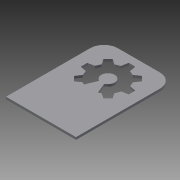
# Autodesk Inventor part: VerticalPiece
Saved by Autodesk Inventor 2014 SP1 (Build 180222100, 222)
## iProperties
Created: 2015-01-04
Part Number: VerticalPiece
Material: Generic
Document SubType Name: Modeling
Designer: Erin
Density: 1 g/cm^3
Appearance: Default
Author: Erin
Autodesk Inventor part; units mm, degrees
ref_plane "YZ Plane" through (0, 0, 0) normal (1, 0, 0) x (0, 1, 0)
ref_plane "XZ Plane" through (0, 0, 0) normal (0, 1, 0) x (-1, 0, 0)
ref_plane "XY Plane" through (0, 0, 0) normal (0, 0, 1) x (1, 0, 0)
sketch "Sketch1" plane through (0, 0, 0) normal (0, 0, 1) x (1, 0, 0)
  line L0 (-15, -18) -> (15, -18)
  line L1 (15, -18) -> (15, 18)
  line L2 (9, 24) -> (-9, 24)
  line L3 (-15, 18) -> (-15, -18)
  arc A0 (-9, 24) -> (-15, 18) centre (-9, 18) ccw
  arc A1 (15, 18) -> (9, 24) centre (9, 18) ccw
  point P0 (0, 0)
  point P1 (15, 24)
  point P2 (-15, 24)
  point P3 (15, 0)
  point P4 (0, 24)
  dimension "d0" = 30
  dimension "d1" = 42
  dimension "d2" = 6
  constraints: 8 end point, 4 point on circle, 4 point on line, 4 tangent, 2 centre point, 2 midpoint, 2 parallel, 1 equal radius, 1 horizontal, 1 horizontal alignment, 1 perpendicular, 1 vertical alignment
  measures "d0" distance of point (-15, 24) point (15, 24)
  measures "d1" distance of point (15, 24) L0.end
  measures "d2" radius of A0
extrude "Extrusion1" add sketch "Sketch1" along normal blind 1
sketch "Sketch2" plane through (0, 0, 0) normal (0, 0, 1) x (1, 0, 0)
  arc A0 (-3.8619, 17.3067) -> (-3.6654, 17.2925) centre (-3.7499, 17.4911) ccw
  line L0 (-3.6654, 17.2925) -> (-1.9114, 18.0105)
  arc A1 (-1.9114, 18.0105) -> (-1.782, 18.1586) centre (-1.9892, 18.209) ccw
  line L1 (-1.782, 18.1586) -> (-1.2951, 20.7754)
  arc A2 (-1.1603, 20.8876) -> (-1.2951, 20.7754) centre (-1.1555, 20.7447) ccw
  line L2 (-1.1603, 20.8876) -> (0.1418, 20.8876)
  arc A3 (3.0232, 10.5703) -> (-2.7384, 10.57) centre (0.1424, 10.5701) ccw
  arc A4 (-2.7384, 10.57) -> (-1.4094, 8.1444) centre (0.1397, 10.5701) ccw
  arc A5 (-1.4094, 8.1444) -> (-1.2693, 8.0371) centre (-0.717, 8.9031) ccw
  line L3 (-1.2693, 8.0371) -> (-1.0511, 7.9035)
  line L4 (-0.9944, 7.7366) -> (-2.8191, 3.3275)
  arc A6 (-2.9648, 3.2741) -> (-2.8191, 3.3275) centre (-2.9158, 3.3658) ccw
  line L5 (-2.9648, 3.2741) -> (-3.8472, 3.7453)
  arc A7 (-3.8472, 3.7453) -> (-4.0418, 3.7399) centre (-3.9398, 3.572) ccw
  line L6 (-4.0418, 3.7399) -> (-6.0484, 2.3626)
  arc A8 (-6.2232, 2.3788) -> (-6.0484, 2.3626) centre (-6.1253, 2.4841) ccw
  line L7 (-6.2232, 2.3788) -> (-8.061, 4.2166)
  arc A9 (-8.0807, 4.3951) -> (-8.061, 4.2166) centre (-7.9596, 4.3181) ccw
  line L8 (-8.0807, 4.3951) -> (-6.6787, 6.4378)
  arc A10 (-6.6787, 6.4378) -> (-6.6624, 6.6306) centre (-6.8628, 6.5504) ccw
  line L9 (-6.6624, 6.6306) -> (-7.436, 8.5631)
  arc A11 (-7.436, 8.5631) -> (-7.581, 8.6886) centre (-7.6302, 8.4854) ccw
  line L10 (-7.581, 8.6886) -> (-10.0488, 9.1479)
  arc A12 (-10.161, 9.2831) -> (-10.0488, 9.1479) centre (-10.0181, 9.2876) ccw
  line L11 (-10.161, 9.2831) -> (-10.1612, 11.8869)
  arc A13 (-10.049, 12.0221) -> (-10.1612, 11.8869) centre (-10.018, 11.8822) ccw
  line L12 (-10.049, 12.0221) -> (-7.5191, 12.4926)
  arc A14 (-7.5191, 12.4926) -> (-7.3693, 12.6214) centre (-7.5703, 12.7036) ccw
  line L13 (-7.3693, 12.6214) -> (-6.5937, 14.4306)
  arc A15 (-6.5937, 14.4306) -> (-6.6058, 14.6262) centre (-6.7865, 14.5168) ccw
  line L14 (-6.6058, 14.6262) -> (-8.0801, 16.7747)
  arc A16 (-8.0639, 16.9496) -> (-8.0801, 16.7747) centre (-7.9592, 16.8517) ccw
  line L15 (-8.0639, 16.9496) -> (-6.2228, 18.7908)
  arc A17 (-6.048, 18.8069) -> (-6.2228, 18.7908) centre (-6.125, 18.6867) ccw
  line L16 (-6.048, 18.8069) -> (-3.8619, 17.3067)
  arc A18 (-0.9944, 7.7366) -> (-1.0511, 7.9035) centre (-1.1231, 7.786) ccw
  line L17 (0.1418, 20.8876) -> (0.1429, 2.0479) construction
  arc A19 (2.0659, 18.1588) -> (2.1953, 18.0107) centre (2.2731, 18.2093) ccw
  line L18 (2.0659, 18.1588) -> (1.5788, 20.7755)
  arc A20 (1.6945, 8.1446) -> (3.0232, 10.5703) centre (0.145, 10.5701) ccw
  arc A21 (1.5544, 8.0373) -> (1.6945, 8.1446) centre (1.002, 8.9032) ccw
  line L19 (1.5544, 8.0373) -> (1.3362, 7.9037)
  line L20 (1.2795, 7.7367) -> (3.1047, 3.3278)
  line L21 (8.3662, 4.3961) -> (6.964, 6.4386)
  arc A22 (8.3466, 4.2175) -> (8.3662, 4.3961) centre (8.2451, 4.319) ccw
  arc A23 (4.3274, 3.7404) -> (4.1328, 3.7458) centre (4.2254, 3.5724) ccw
  line L22 (3.2504, 3.2745) -> (4.1328, 3.7458)
  arc A24 (3.1047, 3.3278) -> (3.2504, 3.2745) centre (3.2014, 3.3662) ccw
  line L23 (4.3274, 3.7404) -> (6.3342, 2.3633)
  arc A25 (6.3342, 2.3633) -> (6.509, 2.3795) centre (6.411, 2.4848) ccw
  line L24 (6.509, 2.3795) -> (8.3466, 4.2175)
  line L25 (10.3336, 12.0232) -> (7.8037, 12.4935)
  arc A26 (10.4458, 11.8881) -> (10.3336, 12.0232) centre (10.3027, 11.8834) ccw
  arc A27 (7.866, 8.6895) -> (7.7211, 8.564) centre (7.9152, 8.4863) ccw
  arc A28 (10.3338, 9.1491) -> (10.446, 9.2843) centre (10.3031, 9.2887) ccw
  line L26 (7.866, 8.6895) -> (10.3338, 9.1491)
  line L27 (6.9477, 6.6314) -> (7.7211, 8.564)
  arc A29 (6.9477, 6.6314) -> (6.964, 6.4386) centre (7.148, 6.5512) ccw
  line L28 (10.446, 9.2843) -> (10.4458, 11.8881)
  arc A30 (3.9494, 17.293) -> (4.1459, 17.3071) centre (4.0339, 17.4915) ccw
  line L29 (3.9494, 17.293) -> (2.1953, 18.0107)
  arc A31 (7.6539, 12.6222) -> (7.8037, 12.4935) centre (7.8549, 12.7045) ccw
  line L30 (7.6539, 12.6222) -> (6.878, 14.4314)
  arc A32 (6.8902, 14.627) -> (6.878, 14.4314) centre (7.0708, 14.5176) ccw
  line L31 (6.8902, 14.627) -> (8.3642, 16.7757)
  arc A33 (8.3642, 16.7757) -> (8.348, 16.9506) centre (8.2433, 16.8527) ccw
  line L32 (1.4439, 20.8877) -> (0.1418, 20.8876)
  arc A34 (1.5788, 20.7755) -> (1.4439, 20.8877) centre (1.4392, 20.7449) ccw
  line L33 (6.3318, 18.8076) -> (4.1459, 17.3071)
  arc A35 (1.3362, 7.9037) -> (1.2795, 7.7367) centre (1.4082, 7.7861) ccw
  line L34 (8.348, 16.9506) -> (6.5066, 18.7915)
  arc A36 (6.5066, 18.7915) -> (6.3318, 18.8076) centre (6.4089, 18.6874) ccw
  point P0 (0, 0)
  point P1 (0.145, 10.5701)
  point P2 (0.145, 10.5701)
  point P3 (0.145, 10.5701)
  dimension "d5" = 18.525
  constraints: 74 point on circle, 71 end point, 54 symmetric about line, 37 centre point, 7 tangent, 1 parallel, 1 perpendicular, 18 other
  measures "d5" distance from line of L23.end L32
extrude "Extrusion2" cut sketch "Sketch2" along normal blind 1
body "Solid1"
